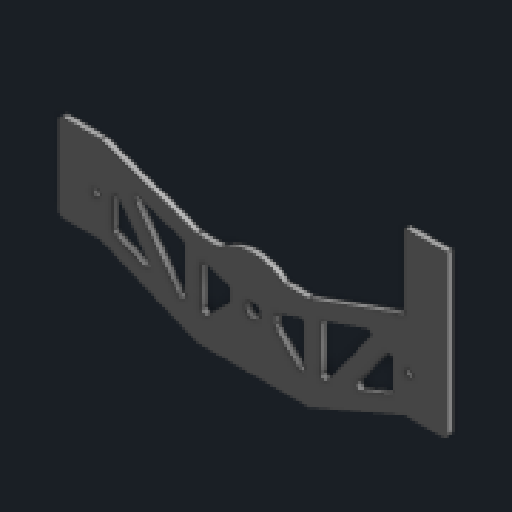
# Autodesk Inventor part: NeckBase
Saved by Autodesk Inventor 2025.2 (Build 292293000, 293)
## iProperties
Created: 2025-08-15
Part Number: NeckBase
Material: Generic
Document SubType Name: Sheet Metal
Designer: valer
Density: 1 g/cm^3
Sheet Metal Rule: Default
Appearance: Default
Author: valer
Autodesk Inventor part; units mm, degrees
ref_plane "YZ Plane" through (0, 0, 0) normal (1, 0, 0) x (0, 1, 0)
ref_plane "XZ Plane" through (0, 0, 0) normal (0, 1, 0) x (-1, 0, 0)
ref_plane "XY Plane" through (0, 0, 0) normal (0, 0, 1) x (1, 0, 0)
sketch "Sketch1" plane through (0, 0, 0) normal (0, 0, 1) x (1, 0, 0)
  arc A0 (-1.9365, 3.5) -> (1.9365, 3.5) centre (0, 0) ccw
  line L0 (1.9365, 3.5) -> (-1.9365, 3.5)
  circle A1 centre (0, 0) radius 19.125 construction
  line L1 (0, -28.5) -> (-28.5, -28.5)
  line L2 (-28.5, -28.5) -> (-77.549, -7.6799)
  line L3 (-77.549, -7.6799) -> (-99.2176, -7.6799)
  line L4 (-99.2176, -7.6799) -> (-99.2176, 36.5969)
  line L5 (-99.2176, 36.5969) -> (-77.549, 36.5969)
  line L6 (-77.549, 36.5969) -> (-28.5, 19.125)
  line L7 (-28.5, 19.125) -> (0, 19.125)
  line L8 (0, -49.1562) -> (0, 95.4371) construction
  line L9 (-28.5, -28.5) -> (-28.5, 19.125) construction
  line L10 (-77.549, -7.6799) -> (-77.549, 36.5969) construction
  circle A2 centre (0, 0) radius 25
  line L11 (28.5, -28.5) -> (77.549, -7.6799)
  line L12 (77.549, -7.6799) -> (99.2176, -7.6799)
  line L13 (99.2176, -7.6799) -> (99.2176, 36.5969)
  line L14 (99.2176, 36.5969) -> (77.549, 36.5969)
  line L15 (77.549, 36.5969) -> (28.5, 19.125)
  line L16 (28.5, 19.125) -> (0, 19.125)
  line L17 (-28.5, 24.5) -> (-28.5, -24.5) construction
  line L18 (-34.5, 12.7699) -> (-34.5, -17.2623)
  line L19 (-34.5, -17.2623) -> (-63.9384, 23.2563)
  line L20 (-48.798, -11.1931) -> (-71.549, 20.1209)
  line L21 (-71.549, 20.1209) -> (-71.549, -1.5359)
  line L22 (-71.549, -1.5359) -> (-48.798, -11.1931)
  line L23 (-34.5, -17.2623) -> (-48.798, -11.1931) construction
  line L24 (-34.5, 12.7699) -> (-63.9384, 23.2563)
  line L25 (34.5, 12.7699) -> (34.5, -17.2623)
  line L26 (34.5, -17.2623) -> (63.9384, 23.2563)
  line L27 (48.798, -11.1931) -> (71.549, 20.1209)
  line L28 (71.549, 20.1209) -> (71.549, -1.5359)
  line L29 (71.549, -1.5359) -> (48.798, -11.1931)
  line L30 (34.5, 12.7699) -> (63.9384, 23.2563)
  line L31 (28.5, -28.5) -> (0, -28.5)
  line L32 (-63.9384, 23.2563) -> (-71.549, 20.1209) construction
  line L33 (99.2176, 36.5969) -> (99.2176, 74.7809)
  line L34 (99.2176, 74.7809) -> (77.549, 74.7809)
  line L35 (77.549, 74.7809) -> (77.549, 36.5969)
  point P0 (-77.549, 14.4585)
  point P1 (16.1008, 19.125)
  point P2 (-16.1008, 19.125)
  dimension "d1" = 50
  dimension "d6" = 6
  dimension "d7" = 6
  dimension "d8" = 8
  dimension "d9" = 8
  dimension "d10" = 8
  dimension "d11" = 36
  dimension "d15" = 15.625
  dimension "d16" = 4
  dimension "d29" = 157
  dimension "d30" = 157
  dimension "d31" = 160.393
  dimension "d32" = 160.393
  dimension "d33" = 49.049
  dimension "d34" = 28.5
  dimension "d35" = 21.6686
  dimension "d36" = 44.2769
  dimension "d37" = 38.1839
  dimension "d38" = 28.5
  dimension "d39" = 5.875
  dimension "d40" = 15.125
  dimension "d41" = 30.0322
  dimension "d42" = 8
  dimension "d43" = 6
  measures "d1" diameter of A2
  measures "d6" distance between parallel lines of L17 L18
  measures "d7" distance from line of point (-77.549, 14.459) L21
  measures "d8" distance between parallel lines of L2 L22
  measures "d9" distance between parallel lines of L6 L24
  measures "d10" distance between parallel lines of L20 L19
  measures "d11" angle of L18 L19
  measures "d15" distance between parallel lines of L16 L0
  measures "d16" radius of A0
  measures "d29" angle of L31 L11
  measures "d30" angle of L2 L1
  measures "d31" angle of L16 L15
  measures "d32" angle of L6 L7
  measures "d33" horizontal distance of L11.start L11.end
  measures "d34" distance of L11.start L1.start
  measures "d35" distance of L11.end L12.end
  measures "d36" distance of L12.end L14.start
  measures "d37" distance of L14.start L33.end
  measures "d38" distance from line of L31 point (0, 0)
  measures "d39" radial gap between concentric circles of A1 A2
  measures "d40" radial gap between concentric circles of A0 A1
  measures "d41" distance of L25.start L25.end
  measures "d42" distance between parallel lines of L26 L27
  measures "d43" distance from line of L11.end L28
extrude "Plate1" add sketch "Sketch1" along normal blind 3.048
fillet "Fillet1" radius 2 9 edges at (99.2176, -7.6799, 1.524) (-99.2176, -7.6799, 1.524) (-99.2176, 36.5969, 1.524) (-28.5, -28.5, 1.524) (28.5, -28.5, 1.524) (-28.5, 19.125, 1.524) (-16.1008, 19.125, 1.524) (16.1008, 19.125, 1.524) (28.5, 19.125, 1.524)
fillet "Fillet2" radius 2 12 edges at (71.549, -1.5359, 1.524) (48.798, -11.1931, 1.524) (34.5, 12.7699, 1.524) (34.5, -17.2623, 1.524) (63.9384, 23.2563, 1.524) (-34.5, -17.2623, 1.524) (-34.5, 12.7699, 1.524) (-63.9384, 23.2563, 1.524) (-48.798, -11.1931, 1.524) (-71.549, -1.5359, 1.524) (-71.549, 20.1209, 1.524) (71.549, 20.1209, 1.524)
sketch "Sketch2" plane through (0, 0, 3.048) normal (0, 0, 1) x (1, 0, 0)
  circle A0 centre (-79.9496, 11.9377) radius 2 projected
  circle A1 centre (79.9496, 11.9377) radius 2 projected
  point P0 (0, 0)
extrude "Cut1" cut sketch "Sketch2" against normal blind 3.048
sketch "Sketch3" plane through (0, 0, 3.048) normal (0, 0, 1) x (1, 0, 0)
  line L0 (26.5, -17.5) -> (11, -2)
  line L1 (11, -2) -> (11, 4.3989)
  line L2 (11, 4.3989) -> (26.5, 9.9202)
  line L3 (26.5, 9.9202) -> (26.5, -17.5)
  line L4 (34.5, -11.1069) -> (34.5, 11.3592) projected
  line L5 (35.8289, 13.2432) -> (57.8509, 21.0878) projected
  line L6 (28.0931, -28.5) -> (-28.0931, -28.5) construction
  line L7 (0, -28.5) -> (0, 3.5) construction
  line L8 (1.9365, 3.5) -> (-1.9365, 3.5) projected
  line L9 (18.1863, -20.5) -> (7.6863, -10)
  line L10 (7.6863, -10) -> (0, -10)
  line L11 (18.1863, -20.5) -> (0, -20.5)
  line L12 (-26.5, -17.5) -> (-11, -2)
  line L13 (-11, -2) -> (-11, 4.3989)
  line L14 (-11, 4.3989) -> (-26.5, 9.9202)
  line L15 (-26.5, 9.9202) -> (-26.5, -17.5)
  line L16 (-18.1863, -20.5) -> (-7.6863, -10)
  line L17 (-7.6863, -10) -> (0, -10)
  line L18 (-18.1863, -20.5) -> (0, -20.5)
  point P0 (0, 0)
  dimension "d19" = 8
  dimension "d20" = 45
  dimension "d21" = 11
  dimension "d22" = 11
  dimension "d23" = 8
  dimension "d24" = 8
  dimension "d25" = 8
  constraints: 30 end point, 6 symmetric about line, 2 midpoint, 2 parallel, 2 perpendicular, 2 point on line, 1 collinear, 1 vertical
  measures "d19" distance between parallel lines of L3 L4
  measures "d20" angle of L0 L3
  measures "d21" distance from line of L6 L0.start
  measures "d22" distance from line of point (0, 0) L1
  measures "d23" distance between parallel lines of L0 L9
  measures "d24" distance between parallel lines of L6 L11
  measures "d25" distance from line of L0.end L10
extrude "Cut2" cut sketch "Sketch3" against normal blind 3.048 contours L0 L1 L2 L3 | L15 L14 L13 L12
fillet "Fillet3" radius 2 8 edges at (-26.5, -17.5, 1.524) (26.5, -17.5, 1.524) (26.5, 9.9202, 1.524) (11, -2, 1.524) (11, 4.3989, 1.524) (-11, -2, 1.524) (-11, 4.3989, 1.524) (-26.5, 9.9202, 1.524)
equation "\"d17\" = Thickness"
equation "\"d26\" = Thickness"
equation "\"d12\" = Thickness"
equation "\"BendRadius\" = Thickness"
equation "\"BendReliefWidth\" = Thickness"
equation "\"BendReliefDepth\" = 0.5 * Thickness"
equation "\"CornerReliefSize\" = 4 * Thickness"
equation "\"MinimumRemnant\" = 2 * Thickness"
equation "\"TransitionRadius\" = BendRadius"
equation "\"JacobiRadiusSize\" = BendRadius"
equation "\"GapSize\" = Thickness"
equation "\"Thickness\" = 3.048"
body "Solid1"
